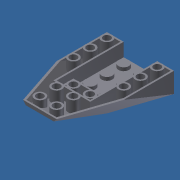
# Autodesk Inventor part: LEGO Brick 4855
Saved by Autodesk Inventor 2011 SP2 (Build 150309200, 309)
## iProperties
Company: Allseas Engineering BV
Created: 2011-09-27
Part Number: LEGO Brick 4855
Cost Center: 0 kg
Material: Steel
Document SubType Name: Modeling
Designer: BvH
Authority: 0 mm^3
Stock Number: =<Filenr>_<Document number>
Density: 7.85 g/cm^3
Act. Code: DW000
SaveDate: 2011-07-28
SaveTime: 18:32
FileName: Standard
TotalMass: 0 kg
TotalVolume: 0 mm^3
Subject: =<Title><TITLE 1_2> <TITLE 2_2>
Author: BvH
Autodesk Inventor part; units mm, degrees
ref_plane "XZ Plane" through (0, 0, 0) normal (0, 1, 0) x (-1, 0, 0)
ref_plane "XY Plane" through (0, 0, 0) normal (0, 0, 1) x (1, 0, 0)
sketch "Sketch1" plane through (0, 0, 0) normal (0, 0, 1) x (1, 0, 0)
  line L0 (0, -33.6) -> (0, 33.6) construction
  line L1 (-22.4, 0) -> (22.4, 0) construction
  line L2 (-16, 24) -> (16, 24)
  line L3 (16, 24) -> (16, 0)
  line L4 (16, 0) -> (8, -24)
  line L5 (8, -24) -> (-8, -24)
  line L6 (-8, -24) -> (-16, 0)
  line L7 (-16, 0) -> (-16, 24)
  line L8 (-8, 24) -> (-8, -8)
  line L9 (-8, -8) -> (8, -8)
  line L10 (8, -8) -> (8, 24)
  line L11 (12, 20) -> (-12, 20) construction
  circle A0 centre (-12, 20) radius 2.5
  circle A1 centre (12, 20) radius 2.5
  line L12 (-4, -12) -> (4, -12) construction
  line L13 (4, -12) -> (4, -20) construction
  line L14 (4, -20) -> (-4, -20) construction
  line L15 (-4, -20) -> (-4, -12) construction
  circle A2 centre (-4, -12) radius 2.5
  circle A3 centre (4, -12) radius 2.5
  circle A4 centre (4, -20) radius 2.5
  circle A5 centre (-4, -20) radius 2.5
  line L16 (-4, 20) -> (4, 20) construction
  circle A6 centre (-4, 20) radius 2.5
  circle A7 centre (4, 20) radius 2.5
  circle A8 centre (4, 4) radius 2.5
  circle A9 centre (-4, 4) radius 2.5
  line L17 (-4, -4) -> (4, -4) construction
  circle A10 centre (-4, -4) radius 2.5
  circle A11 centre (4, -4) radius 2.5
  line L18 (-8, 0) -> (8, 0)
  line L19 (-4, 4) -> (-4, 20) construction
  line L20 (4, 4) -> (4, 20) construction
  circle A12 centre (-4, 12) radius 2.5
  circle A13 centre (4, 12) radius 2.5
  line L21 (-12, 4) -> (12, 4) construction
  line L22 (-12, 12) -> (12, 12) construction
  circle A14 centre (-12, 4) radius 2.5
  circle A15 centre (-12, 12) radius 2.5
  circle A16 centre (12, 12) radius 2.5
  circle A17 centre (12, 4) radius 2.5
  point P0 (0, -24)
  point P1 (0, 24)
  point P2 (0, -8)
  point P3 (0, -20)
  point P4 (0, 20)
  point P5 (8, 8)
  point P6 (0, 0)
  point P7 (0, -4)
  point P8 (0, 4)
  point P9 (0, 12)
  dimension "d2" = 32
  dimension "d3" = 16
  dimension "d4" = 24
  dimension "d5" = 24
  dimension "d7" = 16
  dimension "d8" = 32
  dimension "d9" = 5
  dimension "d10" = 24
  dimension "d11" = 4
  dimension "d12" = 8
  dimension "d13" = 4
  dimension "d14" = 8
  dimension "d15" = 8
  dimension "d55" = 4
  dimension "d56" = 4
  dimension "d57" = 8
  dimension "d58" = 8
  constraints: 42 end point, 18 centre point, 17 equal radius, 15 coincident, 14 midpoint, 10 horizontal, 7 point on line, 6 vertical, 5 parallel, 1 perpendicular, 9 other
  measures "d2" distance between parallel lines of L3 L7
  measures "d3" distance of L4.end L5.end
  measures "d4" distance of L2.end L3.end
  measures "d5" vertical distance of L3.end L4.end
  measures "d7" distance between parallel lines of L10 L8
  measures "d8" distance between parallel lines of L9 L2
  measures "d9" diameter of A0
  measures "d10" distance of L11.start L11.end
  measures "d11" distance between parallel lines of L11 L2
  measures "d12" distance between parallel lines of L13 L15
  measures "d13" distance between parallel lines of L14 L5
  measures "d14" distance between parallel lines of L12 L14
  measures "d15" distance of L16.start L16.end
  measures "d55" distance from line of L20.start L18
  measures "d56" distance between parallel lines of L9 L17
  measures "d57" distance between parallel lines of L9 L18
  measures "d58" distance between parallel lines of L11 L22
extrude "Extrusion1" add sketch "Sketch1" along normal blind 9.6 contours L2 L8 L9 L10 L3 L4 L5 L6 L7 | A0 | A1 | A2 | A3 | A4 | A5 | A14 | A15 | A16 | A17
extrude "Extrusion6" add sketch "Sketch1" along normal blind 3.2 separate body contours L2 L10 L18 L8 | A6 | A7 | A8 | A9 | A12 | A13
extrude "Extrusion7" add sketch "Sketch1" along normal blind 6.4 separate body contours L18 L10 L9 L8 | A10 | A11
extrude "Extrusion8" add sketch "Sketch1" along normal blind 11.2 separate body contours A0 | A1 | A2 | A3 | A4 | A5 | A14 | A15 | A16 | A17
extrude "Extrusion9" add sketch "Sketch1" along normal blind 4.8 separate body contours A6 | A7 | A8 | A9 | A12 | A13
extrude "Extrusion10" add sketch "Sketch1" along normal blind 8 separate body contours A10 | A11
sketch "Sketch2" plane through (0, 0, 0) normal (1, 0, 0) x (0, 1, 0)
  line L0 (-24, 0) -> (-24, 9.6) projected
  line L1 (0, 0) -> (0, 9.6) construction
  line L2 (24, 0) -> (24, 9.6) projected
  line L3 (24, 0) -> (0, 0)
  line L4 (-24, 8) -> (0, 0)
  line L5 (24, 9.6) -> (-24, 9.6)
  dimension "d40" = 1.6
  constraints: 6 end point, 2 horizontal, 1 point on line
  measures "d40" distance from line of L4.start L5
ref_plane "Work Plane1" through (0, -24, 8) normal (0, -0.3162278, -0.9486833) x (0, 0.9486833, -0.3162278)
split "Split2" plane through (0, -24, 8) removes the side toward (0, -0.3162278, -0.9486833) bodies 1
split "Split3" plane through (0, -24, 8) removes the side toward (0, -0.3162278, -0.9486833) bodies 4
split "Split4" plane through (0, -24, 8) removes the side toward (0, -0.3162278, -0.9486833) bodies 3
split "Split5" plane through (0, -24, 8) removes the side toward (0, -0.3162278, -0.9486833) bodies 6
sketch "Sketch3" plane through (0, 0, 0) normal (0, 1, 0) x (-1, 0, 0)
  line L0 (-16, 0) -> (-16, 9.6) projected
  line L1 (16, 0) -> (16, 9.6) projected
  line L2 (8, 0) -> (8, 9.6) construction
  line L3 (-8, 0) -> (-8, 9.6) construction
  line L4 (-8, 0) -> (8, 0)
  line L5 (8, 0) -> (16, 8)
  line L6 (-8, 0) -> (-16, 8)
  line L7 (-16, 9.6) -> (16, 9.6)
  line L8 (-16, 8) -> (16, 8) construction
  dimension "d41" = 1.6
  constraints: 10 end point, 2 horizontal, 2 point on line, 1 parallel
  measures "d41" distance between parallel lines of L8 L7
ref_plane "Work Plane2" through (16, 24, 0) normal (0.7442084, -0.2480695, -0.6201737) x (0, -0.9284767, 0.3713907)
ref_plane "Work Plane3" through (-16, 24, 0) normal (0.7442084, 0.2480695, 0.6201737) x (0, -0.9284767, 0.3713907)
split "Split6" plane through (16, 24, 0) removes the side toward (0.7442084, -0.2480695, -0.6201737) bodies 1
split "Split7" plane through (16, 24, 0) removes the side toward (0.7442084, -0.2480695, -0.6201737) bodies 4
split "Split8" plane through (-16, 24, 0) removes the side toward (-0.7442084, -0.2480695, -0.6201737) bodies 1
split "Split9" plane through (-16, 24, 0) removes the side toward (-0.7442084, -0.2480695, -0.6201737) bodies 4
split "Split10" plane through (16, 24, 0) removes the side toward (0.7442084, -0.2480695, -0.6201737) bodies 3
split "Split11" plane through (-16, 24, 0) removes the side toward (-0.7442084, -0.2480695, -0.6201737) bodies 3
shell "Shell1" thickness 0.8 removed faces 1 at (2.6667, -18.6667, 9.6) bodies 1
shell "Shell2" thickness 0.8 removed faces 10 at (-3.5191, -21.5312, 11.2) at (-4.7379, -12.3873, 11.2) at (4.7621, -12.5867, 11.2) at (3.3762, -20.5526, 11.2) at (-12.6238, 19.4474, 11.2) at (11.3762, 19.4474, 11.2) at (12.8091, 11.4249, 11.2) at (12.2955, 4.7792, 11.2) at (-11.7045, 4.7792, 11.2) at (-11.1909, 11.4249, 11.2) bodies 4
shell "Shell3" thickness 0.8 removed faces 1 at (-2.6667, -2.6667, 6.4) bodies 3
shell "Shell4" thickness 0.8 removed faces 2 at (-4.2955, -3.2208, 8) at (3.7045, -3.2208, 8) bodies 6
combine bodies "Combine1" operation type add bodies to combine 1 2 3 4 5 6
sketch "Sketch5" plane through (16, 24, 0) normal (0, 0, -1) x (-1, 0, 0)
  circle A0 centre (20, -4) radius 2.5 construction
  circle A1 centre (12, -20) radius 2.5 construction
  line L0 (9.5, -22.5) -> (22.5, -22.5)
  line L1 (22.5, -22.5) -> (22.5, -1.5)
  line L2 (22.5, -1.5) -> (9.5, -1.5)
  line L3 (9.5, -1.5) -> (9.5, -22.5)
  constraints: 8 end point, 4 tangent, 2 parallel, 1 horizontal, 1 perpendicular
extrude "Extrusion13" cut sketch "Sketch5" against normal blind 1.6 bodies 1
body "Solid1"
